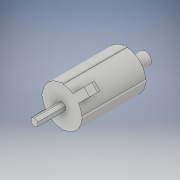
# Autodesk Inventor part: eix bobina
Saved by Autodesk Inventor 2019 (Build 230136000, 136)
## iProperties
Created: 2018-08-16
Part Number: eix bobina
Material: Genérico
Document SubType Name: Modeling
Designer: Albert Garangou Culebras
Density: 1 g/cm^3
Appearance: Valor por defecto
Author: Albert Garangou Culebras
Autodesk Inventor part; units mm, degrees
ref_plane "YZ Plane" through (0, 0, 0) normal (1, 0, 0) x (0, 1, 0)
ref_plane "XZ Plane" through (0, 0, 0) normal (0, 1, 0) x (-1, 0, 0)
ref_plane "XY Plane" through (0, 0, 0) normal (0, 0, 1) x (1, 0, 0)
sketch "Boceto1" plane through (0, 0, 0) normal (0, 0, 1) x (1, 0, 0)
  circle A0 centre (0, 0) radius 25
  line L0 (0, 25) -> (0, 26.5)
  arc A1 (1.4993, 24.955) -> (0, 26.5) centre (0, 25) ccw
  arc A2 (0, 26.5) -> (-1.4993, 24.955) centre (0, 25) ccw
  line L1 (0, -25) -> (0, -26.5)
  arc A3 (0, -26.5) -> (1.4993, -24.955) centre (0, -25) ccw
  arc A4 (-1.4993, -24.955) -> (0, -26.5) centre (0, -25) ccw
  line L2 (25, 0) -> (26.5, 0)
  line L3 (-25, 0) -> (-26.5, 0)
  arc A5 (-24.955, 1.4993) -> (-24.955, -1.4993) centre (-25, 0) ccw
  arc A6 (24.955, -1.4993) -> (24.955, 1.4993) centre (25, 0) ccw
  dimension "d0" = 50
  dimension "d1" = 1.5
  dimension "d2" = 1.5
  dimension "d4" = 1.5
  constraints: 14 point on circle, 8 end point, 6 centre point, 6 coincident, 2 horizontal, 2 vertical, 15 other
  measures "d1" distance of L0.start L0.end
  measures "d2" distance of L1.start L1.end
  measures "d4" distance of L3.start L3.end
extrude "Extrusión1" add sketch "Boceto1" along normal blind 81
sketch "Boceto2" plane through (0, 0, 81) normal (0, 0, 1) x (1, 0, 0)
  line L0 (0, 5) -> (4.3301, 2.5)
  line L1 (4.3301, 2.5) -> (4.3301, -2.5)
  line L2 (4.3301, -2.5) -> (0, -5)
  line L3 (0, -5) -> (-4.3301, -2.5)
  line L4 (-4.3301, -2.5) -> (-4.3301, 2.5)
  line L5 (-4.3301, 2.5) -> (0, 5)
  point P0 (0, 0)
  point P1 (0, 0)
  constraints: 12 end point, 1 coincident, 13 other
extrude "Extrusión2" add sketch "Boceto2" along normal blind 35
sketch "Boceto3" plane through (0, 0, 81) normal (0, 0, 1) x (1, 0, 0)
  arc A0 (24.955, 1.4993) -> (1.4993, 24.955) centre (0, 0) ccw projected
  arc A1 (24.955, 1.4993) -> (1.4993, 24.955) centre (0, 0) ccw
  line L0 (17.6777, 17.6777) -> (0, 0)
  line L1 (17.6777, 17.6777) -> (13.8063, 20.8419)
  line L2 (17.6777, 17.6777) -> (20.8419, 13.8063)
  line L3 (20.8419, 13.8063) -> (27.9483, 20.8419)
  line L4 (13.8063, 20.8419) -> (20.8419, 27.9483)
  line L5 (20.8419, 27.9483) -> (27.9483, 20.8419)
  dimension "d9" = 5
  dimension "d10" = 5
  dimension "d12" = 10
  dimension "d13" = 10
  constraints: 12 end point, 7 point on circle, 1 centre point, 1 coincident
  measures "d9" distance of L0.start L1.end
  measures "d10" distance of L2.start L2.end
  measures "d12" distance of L2.end L3.end
  measures "d13" distance of L1.end L4.end
extrude "Extrusión3" add sketch "Boceto3" against normal blind 10 contours A0 L4 L5 L3
sketch "Boceto4" plane through (27.9483, 20.8419, 71) normal (0.7071068, 0.7071068, 0) x (-0.7071068, 0.7071068, 0)
  line L0 (9.9999, 0) -> (10.0499, 0) projected
  line L1 (0.05, 10) -> (-11.5607, 10) projected
  line L2 (10.0499, 0) -> (0.05, 0)
  line L3 (0.05, 0) -> (0.05, 10)
  line L4 (0.05, 10) -> (10.0499, 10)
  line L5 (10.0499, 10) -> (10.0499, 0)
  point P0 (5.0249, -71)
  constraints: 8 end point, 2 parallel, 1 horizontal, 1 perpendicular
extrude "Extrusión4" add sketch "Boceto4" along normal blind 10
sketch "Boceto5" plane through (0, 0, 71) normal (0, 0, -1) x (-1, 0, 0)
  line L0 (-34.984, 27.9484) -> (-27.913, 35.0193) projected
  line L1 (-27.9661, 34.9662) -> (-34.984, 27.9484)
  line L2 (-34.984, 27.9484) -> (-27.9484, 20.842)
  line L3 (-20.8419, 27.9483) -> (-27.913, 35.0193) projected
  line L4 (-27.913, 35.0193) -> (-20.8419, 27.9483)
  line L5 (-20.8419, 13.8063) -> (-27.9483, 20.8419) projected
  line L6 (-20.8419, 27.9483) -> (-27.9483, 20.8419)
  line L7 (-20.8419, 27.9483) -> (-13.8063, 20.8419) projected
  line L8 (-20.8419, 27.9483) -> (-27.913, 35.0193)
  line L9 (-27.913, 35.0193) -> (-34.984, 27.9484)
  line L10 (-27.9129, 20.8773) -> (-34.984, 27.9484) projected
  line L11 (-27.9483, 20.8419) -> (-34.984, 27.9484)
  line L12 (-27.9129, 20.8773) -> (-20.8419, 27.9483)
  point P0 (0, 0)
  dimension "d18" = 10
  dimension "d19" = 10
  constraints: 16 end point, 4 collinear, 2 point on line, 1 perpendicular
  measures "d18" distance of L0.start L2.end
  measures "d19" distance of L0.end L3.start
extrude "Extrusión5" add sketch "Boceto5" along normal blind 10 contours L0 L3 L6 L10
sketch "Boceto6" plane through (27.9129, 20.8773, 81) normal (0.7071068, -0.7071068, 0) x (-0.7071068, -0.7071068, 0)
  line L0 (0, 10) -> (0, 20) projected
  line L1 (-10, 10) -> (0, 20)
  line L2 (-10, 20) -> (0, 20) projected
  line L3 (-10, 10) -> (-10, 20)
  line L4 (-10, 20) -> (0, 20)
  point P0 (34.4999, 81)
  constraints: 6 end point, 1 collinear, 1 vertical
extrude "Extrusión6" cut sketch "Boceto6" against normal blind 13.25
sketch "Boceto7" plane through (0, 0, 81) normal (0, 0, 1) x (1, 0, 0)
  arc A0 (-24.955, -1.4993) -> (-1.8412, -24.9321) centre (0, 0) ccw
  line L0 (0, 0) -> (-17.7984, -17.5561)
  arc A1 (-24.955, -1.4993) -> (-1.4993, -24.955) centre (0, 0) ccw projected
  line L1 (-17.7984, -17.5561) -> (-13.9488, -20.7468)
  line L2 (-17.7984, -17.5561) -> (-20.936, -13.6632)
  arc A2 (20.8419, 13.8063) -> (13.8063, 20.8419) centre (0, 0) ccw projected
  line L3 (13.8063, 20.8419) -> (-20.936, -13.6632)
  arc A3 (24.955, 1.4993) -> (20.8419, 13.8063) centre (0, 0) ccw projected
  line L4 (20.8419, 13.8063) -> (-13.9488, -20.7468)
  line L5 (-20.936, -13.6632) -> (-35.1944, -27.6882)
  line L6 (-13.9488, -20.7468) -> (-28.1875, -34.7917)
  line L7 (-28.1875, -34.7917) -> (-35.1944, -27.6882)
  dimension "d24" = 5
  dimension "d25" = 5
  dimension "d29" = 20
  dimension "d30" = 20
  constraints: 16 end point, 6 point on circle, 1 centre point, 1 coincident, 1 perpendicular
  measures "d24" distance of L0.end L1.end
  measures "d25" distance of L0.end L2.end
  measures "d29" distance of L2.end L5.end
  measures "d30" distance of L1.end L6.end
extrude "Extrusión7" add sketch "Boceto7" against normal blind 10 contours A0 L6 L7 L5
sketch "Boceto8" plane through (-20.936, -13.6632, 81) normal (-0.7012491, 0.7129163, 0) x (0.7129163, 0.7012491, 0)
  line L0 (-20, 10) -> (0, 10) projected
  line L1 (-10, 10) -> (-10, 20)
  line L2 (-10, 20) -> (-20, 10)
  line L3 (-10, 10) -> (-20, 10)
  point P0 (24.5069, 81)
  dimension "d33" = 10
  constraints: 6 end point, 1 collinear, 1 midpoint, 1 vertical
  measures "d33" distance of L1.start L1.end
extrude "Extrusión8" add sketch "Boceto8" against normal blind 10
sketch "Boceto10" plane through (0, 0, 0) normal (0, 0, -1) x (-1, 0, 0)
  circle A0 centre (0, 0) radius 7.5
  dimension "d37" = 15
  constraints: 1 centre point, 1 coincident
  measures "d37" diameter of A0
extrude "Extrusión9" add sketch "Boceto10" along normal blind 25
